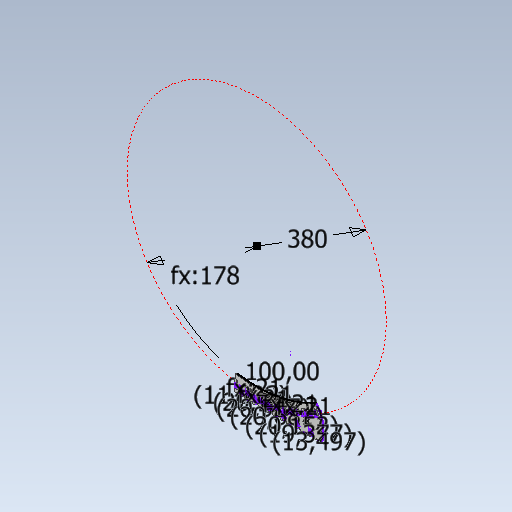
# Autodesk Inventor part: keywell_support-back
Saved by Autodesk Inventor 2020.1 (Build 241239000, 239)
## iProperties
Created: 2019-06-30
Part Number: keywell_support-back
Material: Acier inoxydable
Document SubType Name: Modeling
Designer: Thibault
Density: 8 g/cm^3
Appearance: Semi-poli
Mass: 13.686 g
Surface Area: 39.9351 cm^2
Volume: 1.71076 cm^3
kws_bp_anchor_dist1: 13,497 mm
kws_bp_anchor_dist2: 19,377 mm
kws_bp_anchor_dist3: 20,152 mm
kws_bp_anchor_dist4: 20,681 mm
kws_bp_anchor_dist5: 20,957 mm
kws_bp_anchor_dist6: 20,990 mm
kws_bp_anchor_dist7: 11,809 mm
Author: Thibault
Autodesk Inventor part; units mm, degrees
ref_plane "YZ Plane" through (0, 0, 0) normal (1, 0, 0) x (0, 1, 0)
ref_plane "XZ Plane" through (0, 0, 0) normal (0, 1, 0) x (-1, 0, 0)
ref_plane "XY Plane" through (0, 0, 0) normal (0, 0, 1) x (1, 0, 0)
sketch "Anchor (screw side)" plane through (0, 0, 0) normal (0, 0, 1) x (1, 0, 0)
  circle A0 centre (93.8994, 50.3042) radius 1.05
  line L0 (90.8494, 51.3542) -> (87.7494, 51.3542)
  line L1 (87.7494, 51.3542) -> (87.7494, 49.2542)
  line L2 (87.7494, 49.2542) -> (90.8494, 49.2542)
  line L3 (90.8494, 49.2542) -> (90.8494, 51.3542)
  line L4 (100.0494, 51.3542) -> (96.9494, 51.3542)
  line L5 (96.9494, 51.3542) -> (96.9494, 49.2542)
  line L6 (96.9494, 49.2542) -> (100.0494, 49.2542)
  line L7 (100.0494, 49.2542) -> (100.0494, 51.3542)
  line L8 (90.8494, 51.3542) -> (96.9494, 49.2542) construction
  line L9 (96.9494, 51.3542) -> (90.8494, 49.2542) construction
  line L10 (85.7494, 53.3542) -> (102.0494, 53.3542) construction
  line L11 (102.0494, 53.3542) -> (102.0494, 47.2542) construction
  line L12 (102.0494, 47.2542) -> (85.7494, 47.2542) construction
  line L13 (85.7494, 47.2542) -> (85.7494, 53.3542) construction
  point P0 (103.5798, 50.1132)
  dimension "d27" = 2.1
  dimension "d28" = 3.1
  dimension "d29" = 2.1
  dimension "slot_distance" = 6.1
  dimension "d34" = 2
  dimension "d35" = 2
  dimension "d36" = 2
  dimension "d37" = 2
  measures "d27" diameter of A0
  measures "d28" distance of L2.end L1.end
  measures "d29" distance of L1.end L0.end
  measures "slot_distance" distance between parallel lines of L5 L3
  measures "d34" distance between parallel lines of L0 L10
  measures "d35" distance between parallel lines of L12 L2
  measures "d36" distance between parallel lines of L11 L7
  measures "d37" distance between parallel lines of L13 L1
sketch "Anchor (nut side)" plane through (0, 0, 0) normal (0, 0, 1) x (1, 0, 0)
  line L0 (11.1, 0) -> (9.1, 0)
  line L1 (9.1, 0) -> (9.1, -2)
  line L2 (9.1, -2) -> (9.9, -2)
  line L3 (9.9, -2) -> (9.9, -4)
  line L4 (6.2, -4) -> (6.2, -2)
  line L5 (6.2, -2) -> (7, -2)
  line L6 (7, -2) -> (7, 0)
  line L7 (7, 0) -> (5, 0)
  line L8 (2, 0) -> (2, 2)
  line L9 (2, 0) -> (3, 0) construction
  line L10 (2, 2) -> (5, 2)
  line L11 (5, 2) -> (5, 0)
  line L12 (11.1, 0) -> (11.1, 2)
  line L13 (11.1, 2) -> (14.1, 2)
  line L14 (14.1, 2) -> (14.1, 0)
  line L15 (0, 0) -> (2, 0)
  line L16 (14.1, 0) -> (16.1, 0)
  line L17 (6.2, -4) -> (7, -4)
  line L18 (9.9, -4) -> (9.1, -4)
  line L19 (7, -4) -> (7, -6.25)
  line L20 (9.1, -4) -> (9.1, -6.25)
  line L21 (7.25, -6.5) -> (8.05, -6.5)
  arc A0 (7, -6.25) -> (7.25, -6.5) centre (7.25, -6.25) ccw
  arc A1 (8.85, -6.5) -> (9.1, -6.25) centre (8.85, -6.25) ccw
  line L22 (8.05, -6.5) -> (8.85, -6.5)
  line L23 (8.05, -3.8983) -> (8.05, -9.959) construction
  point P0 (9.1321, -0.6227)
  point P1 (7, -6.5)
  point P2 (9.1, -6.5)
  dimension "d3" = 2
  dimension "d7" = 6.1
  dimension "d10" = 2
  dimension "d11" = 2
  dimension "d12" = 0.8
  dimension "d13" = 2
  dimension "d14" = 0.8
  dimension "d15" = 2.1
  dimension "d18" = 2
  dimension "d19" = 0.8
  dimension "d20" = 0.8
  dimension "d21" = 2.5
  dimension "d22" = 2.5
  dimension "d23" = 2.1
  dimension "d38" = 2
  dimension "d39" = 0.25
  dimension "d120" = 3
  measures "d3" distance of point (0, 0) L8.start
  measures "d7" distance of L7.end L0.start
  measures "d10" distance of L0.start L0.end
  measures "d11" distance of L0.end L1.end
  measures "d12" distance of L1.end L2.end
  measures "d13" distance of L2.end L3.end
  measures "d14" distance of L4.end L5.end
  measures "d15" distance of L6.end L0.end
  measures "d18" distance of L14.end point (16.1, 0)
  measures "d19" distance of L4.start L17.end
  measures "d20" distance of L3.end L18.end
  measures "d21" distance of L17.end point (7, -6.5)
  measures "d22" distance of L18.end point (9.1, -6.5)
  measures "d23" distance of L17.end L18.end
  measures "d38" distance of the line from the sketch origin of L10
  measures "d39" radius of A0
  measures "d120" distance of L8.end L10.end
sketch "Screwless anchor (male)" plane through (0, 0, 0) normal (0, 0, 1) x (1, 0, 0)
  line L0 (2, 0) -> (2, 2)
  line L1 (2, 0) -> (3, 0) construction
  line L2 (2, 2) -> (5, 2)
  line L3 (5, 2) -> (5, 0)
  line L4 (11.1, 0) -> (11.1, 2)
  line L5 (11.1, 2) -> (14.1, 2)
  line L6 (14.1, 2) -> (14.1, 0)
  line L7 (0, 0) -> (2, 0)
  line L8 (14.1, 0) -> (16.1, 0)
  line L9 (5, 0) -> (11.1, 0)
  point P0 (9.1321, -0.6227)
  dimension "d81" = 2
  dimension "d83" = 6.1
  dimension "d92" = 2
  dimension "d100" = 2
  dimension "d119" = 3
  measures "d81" distance of L7.start L0.start
  measures "d83" distance of L3.end L4.start
  measures "d92" distance of L6.end L8.end
  measures "d100" distance between parallel lines of L7 L2
  measures "d119" distance of L0.end L2.end
sketch "Screwless anchor (female)" plane through (0, 0, 0) normal (0, 0, 1) x (1, 0, 0)
  line L0 (91.7814, 51.7592) -> (88.6814, 51.7592)
  line L1 (88.6814, 51.7592) -> (88.6814, 49.6592)
  line L2 (88.6814, 49.6592) -> (91.7814, 49.6592)
  line L3 (91.7814, 49.6592) -> (91.7814, 51.7592)
  line L4 (100.9814, 51.7592) -> (97.8814, 51.7592)
  line L5 (97.8814, 51.7592) -> (97.8814, 49.6592)
  line L6 (97.8814, 49.6592) -> (100.9814, 49.6592)
  line L7 (100.9814, 49.6592) -> (100.9814, 51.7592)
  line L8 (86.6814, 53.7592) -> (102.9814, 53.7592) construction
  line L9 (102.9814, 53.7592) -> (102.9814, 47.6592) construction
  line L10 (102.9814, 47.6592) -> (86.6814, 47.6592) construction
  line L11 (86.6814, 47.6592) -> (86.6814, 53.7592) construction
  point P0 (103.5798, 50.1132)
  dimension "d106" = 3.1
  dimension "d107" = 2.1
  dimension "d108" = 3.1
  dimension "d109" = 6.1
  dimension "d110" = 2
  dimension "d111" = 2
  dimension "d112" = 2
  dimension "d113" = 2
  measures "d106" distance of L2.end L1.end
  measures "d107" distance of L1.end L0.end
  measures "d108" distance of L6.end L5.end
  measures "d109" distance between parallel lines of L5 L3
  measures "d110" distance between parallel lines of L0 L8
  measures "d111" distance between parallel lines of L10 L2
  measures "d112" distance between parallel lines of L9 L7
  measures "d113" distance between parallel lines of L11 L1
sketch "Anchor" plane through (0, 0, 0) normal (0, 0, 1) x (1, 0, 0)
  line L0 (-55.968, -124.6471) -> (-43.668, -138.5471) construction
  line L1 (-43.668, -124.6471) -> (-55.968, -138.5471) construction
  line L2 (-49.818, -129.7478) -> (-49.818, -133.4207) construction
  circle A0 centre (-49.818, -123.5971) radius 1.05
  line L3 (-52.868, -122.5471) -> (-55.968, -122.5471)
  line L4 (-55.968, -122.5471) -> (-55.968, -124.6471)
  line L5 (-55.968, -124.6471) -> (-52.868, -124.6471)
  line L6 (-52.868, -124.6471) -> (-52.868, -122.5471)
  line L7 (-43.668, -122.5471) -> (-46.768, -122.5471)
  line L8 (-46.768, -122.5471) -> (-46.768, -124.6471)
  line L9 (-46.768, -124.6471) -> (-43.668, -124.6471)
  line L10 (-43.668, -124.6471) -> (-43.668, -122.5471)
  line L11 (-52.868, -122.5471) -> (-46.768, -124.6471) construction
  line L12 (-46.768, -122.5471) -> (-52.868, -124.6471) construction
  line L13 (-57.968, -120.5471) -> (-41.668, -120.5471) construction
  line L14 (-41.668, -120.5471) -> (-41.668, -126.6471) construction
  line L15 (-41.668, -126.6471) -> (-57.968, -126.6471) construction
  line L16 (-57.968, -126.6471) -> (-57.968, -120.5471) construction
  circle A1 centre (-49.818, -139.5971) radius 1.05
  line L17 (-52.868, -138.5471) -> (-55.968, -138.5471)
  line L18 (-55.968, -138.5471) -> (-55.968, -140.6471)
  line L19 (-55.968, -140.6471) -> (-52.868, -140.6471)
  line L20 (-52.868, -140.6471) -> (-52.868, -138.5471)
  line L21 (-43.668, -138.5471) -> (-46.768, -138.5471)
  line L22 (-46.768, -138.5471) -> (-46.768, -140.6471)
  line L23 (-46.768, -140.6471) -> (-43.668, -140.6471)
  line L24 (-43.668, -140.6471) -> (-43.668, -138.5471)
  line L25 (-52.868, -138.5471) -> (-46.768, -140.6471) construction
  line L26 (-46.768, -138.5471) -> (-52.868, -140.6471) construction
  line L27 (-57.968, -136.5471) -> (-41.668, -136.5471) construction
  line L28 (-41.668, -136.5471) -> (-41.668, -142.6471) construction
  line L29 (-41.668, -142.6471) -> (-57.968, -142.6471) construction
  line L30 (-57.968, -142.6471) -> (-57.968, -136.5471) construction
  point P0 (-66.8969, -206.6558)
  point P1 (-49.818, -123.5971)
  point P2 (-49.818, -139.5971)
  dimension "d161" = 13.9
sketch "Esquisse2" plane through (0, 0, 0) normal (0, 0, 1) x (1, 0, 0)
  circle A0 centre (0, 0) radius 190 construction
  arc A1 (-29.069, -175.6103) -> (87.3778, -155.0778) centre (0, 0) ccw
  line L0 (-31.1541, -195.9973) -> (-29.069, -175.6103)
  line L1 (49.6599, -108.8996) -> (49.6599, -114.6687) construction
  line L2 (96.3099, -173.5221) -> (96.3099, -198.7774)
  line L3 (-31.1541, -195.9973) -> (-31.1541, -198.7774)
  line L4 (30.8562, -181.468) -> (33.0699, -181.0776) construction
  line L5 (87.3778, -155.0778) -> (96.3099, -173.5221)
  line L6 (-27.395, -198.7774) -> (-31.1541, -198.7774)
  line L7 (-11.295, -198.7774) -> (-6.4051, -198.7774)
  line L8 (9.6949, -198.7774) -> (14.552, -198.7774)
  line L9 (30.652, -198.7774) -> (35.233, -198.7774)
  line L10 (51.333, -198.7774) -> (55.3852, -198.7774)
  line L11 (71.4852, -198.7774) -> (74.7625, -198.7774)
  line L12 (90.8625, -198.7774) -> (96.3099, -198.7774)
  line L13 (28.7711, -181.7178) -> (16.433, -195.584) construction
  line L14 (30.2343, -193.9304) -> (14.9698, -183.3713) construction
  line L15 (24.4382, -188.4309) -> (20.7913, -188.8678) construction
  circle A2 centre (30.5452, -187.6992) radius 1.05
  line L16 (31.2249, -184.546) -> (30.8562, -181.468)
  line L17 (30.8562, -181.468) -> (28.7711, -181.7178)
  line L18 (28.7711, -181.7178) -> (29.1398, -184.7958)
  line L19 (29.1398, -184.7958) -> (31.2249, -184.546)
  line L20 (32.3193, -193.6806) -> (31.9506, -190.6026)
  line L21 (31.9506, -190.6026) -> (29.8655, -190.8525)
  line L22 (29.8655, -190.8525) -> (30.2343, -193.9304)
  line L23 (30.2343, -193.9304) -> (32.3193, -193.6806)
  line L24 (31.2249, -184.546) -> (29.8655, -190.8525) construction
  line L25 (31.9506, -190.6026) -> (29.1398, -184.7958) construction
  line L26 (32.604, -179.2443) -> (34.5431, -195.4285) construction
  line L27 (34.5431, -195.4285) -> (28.4864, -196.1542) construction
  line L28 (28.4864, -196.1542) -> (26.5474, -179.9699) construction
  line L29 (26.5474, -179.9699) -> (32.604, -179.2443) construction
  circle A3 centre (14.6588, -189.6025) radius 1.05
  line L30 (15.3385, -186.4493) -> (14.9698, -183.3713)
  line L31 (14.9698, -183.3713) -> (12.8847, -183.6211)
  line L32 (12.8847, -183.6211) -> (13.2535, -186.6991)
  line L33 (13.2535, -186.6991) -> (15.3385, -186.4493)
  line L34 (16.433, -195.584) -> (16.0642, -192.506)
  line L35 (16.0642, -192.506) -> (13.9791, -192.7558)
  line L36 (13.9791, -192.7558) -> (14.3479, -195.8338)
  line L37 (14.3479, -195.8338) -> (16.433, -195.584)
  line L38 (15.3385, -186.4493) -> (13.9791, -192.7558) construction
  line L39 (16.0642, -192.506) -> (13.2535, -186.6991) construction
  line L40 (16.7177, -181.1476) -> (18.6567, -197.3318) construction
  line L41 (18.6567, -197.3318) -> (12.6, -198.0575) construction
  line L42 (12.6, -198.0575) -> (10.661, -181.8732) construction
  line L43 (10.661, -181.8732) -> (16.7177, -181.1476) construction
  line L44 (86.3871, -162.4389) -> (79.2379, -179.5675) construction
  line L45 (91.7481, -173.5091) -> (73.8769, -168.4973) construction
  line L46 (84.4769, -170.1971) -> (81.1712, -171.798) construction
  circle A4 centre (90.0126, -167.5164) radius 1.05
  line L47 (89.6283, -164.3137) -> (88.2771, -161.5236)
  line L48 (88.2771, -161.5236) -> (86.3871, -162.4389)
  line L49 (86.3871, -162.4389) -> (87.7382, -165.2289)
  line L50 (87.7382, -165.2289) -> (89.6283, -164.3137)
  line L51 (93.6381, -172.5938) -> (92.287, -169.8038)
  line L52 (92.287, -169.8038) -> (90.397, -170.7191)
  line L53 (90.397, -170.7191) -> (91.7481, -173.5091)
  line L54 (91.7481, -173.5091) -> (93.6381, -172.5938)
  line L55 (89.6283, -164.3137) -> (90.397, -170.7191) construction
  line L56 (92.287, -169.8038) -> (87.7382, -165.2289) construction
  line L57 (89.2055, -158.8519) -> (96.3099, -173.5221) construction
  line L58 (96.3099, -173.5221) -> (90.8198, -176.1808) construction
  line L59 (90.8198, -176.1808) -> (83.7154, -161.5106) construction
  line L60 (83.7154, -161.5106) -> (89.2055, -158.8519) construction
  circle A5 centre (75.6124, -174.49) radius 1.05
  line L61 (75.228, -171.2873) -> (73.8769, -168.4973)
  line L62 (73.8769, -168.4973) -> (71.9868, -169.4126)
  line L63 (71.9868, -169.4126) -> (73.338, -172.2026)
  line L64 (73.338, -172.2026) -> (75.228, -171.2873)
  line L65 (79.2379, -179.5675) -> (77.8867, -176.7774)
  line L66 (77.8867, -176.7774) -> (75.9967, -177.6927)
  line L67 (75.9967, -177.6927) -> (77.3478, -180.4828)
  line L68 (77.3478, -180.4828) -> (79.2379, -179.5675)
  line L69 (75.228, -171.2873) -> (75.9967, -177.6927) construction
  line L70 (77.8867, -176.7774) -> (73.338, -172.2026) construction
  line L71 (74.8052, -165.8255) -> (81.9096, -180.4958) construction
  line L72 (81.9096, -180.4958) -> (76.4195, -183.1545) construction
  line L73 (76.4195, -183.1545) -> (69.3151, -168.4843) construction
  line L74 (69.3151, -168.4843) -> (74.8052, -165.8255) construction
  line L75 (-5.2516, -196.2028) -> (8.5414, -183.7829) construction
  line L76 (-5.358, -183.9033) -> (8.6479, -196.0825) construction
  line L77 (-0.2043, -190.0089) -> (3.4685, -189.9771) construction
  circle A6 centre (-6.3548, -190.0621) radius 1.05
  line L78 (-7.3783, -193.1211) -> (-7.3515, -196.221)
  line L79 (-7.3515, -196.221) -> (-5.2516, -196.2028)
  line L80 (-5.2516, -196.2028) -> (-5.2784, -193.1029)
  line L81 (-5.2784, -193.1029) -> (-7.3783, -193.1211)
  line L82 (-7.458, -183.9215) -> (-7.4311, -187.0213)
  line L83 (-7.4311, -187.0213) -> (-5.3312, -187.0032)
  line L84 (-5.3312, -187.0032) -> (-5.358, -183.9033)
  line L85 (-5.358, -183.9033) -> (-7.458, -183.9215)
  line L86 (-7.3783, -193.1211) -> (-5.3312, -187.0032) construction
  line L87 (-7.4311, -187.0213) -> (-5.2784, -193.1029) construction
  line L88 (-9.3341, -198.2382) -> (-9.4752, -181.9389) construction
  line L89 (-9.4752, -181.9389) -> (-3.3754, -181.886) construction
  line L90 (-3.3754, -181.886) -> (-3.2343, -198.1854) construction
  line L91 (-3.2343, -198.1854) -> (-9.3341, -198.2382) construction
  circle A7 centre (9.6446, -189.9236) radius 1.05
  line L92 (8.6211, -192.9826) -> (8.6479, -196.0825)
  line L93 (8.6479, -196.0825) -> (10.7478, -196.0643)
  line L94 (10.7478, -196.0643) -> (10.721, -192.9644)
  line L95 (10.721, -192.9644) -> (8.6211, -192.9826)
  line L96 (8.5414, -183.7829) -> (8.5683, -186.8828)
  line L97 (8.5683, -186.8828) -> (10.6682, -186.8646)
  line L98 (10.6682, -186.8646) -> (10.6414, -183.7648)
  line L99 (10.6414, -183.7648) -> (8.5414, -183.7829)
  line L100 (8.6211, -192.9826) -> (10.6682, -186.8646) construction
  line L101 (8.5683, -186.8828) -> (10.721, -192.9644) construction
  line L102 (6.6653, -198.0997) -> (6.5242, -181.8003) construction
  line L103 (6.5242, -181.8003) -> (12.624, -181.7475) construction
  line L104 (12.624, -181.7475) -> (12.7651, -198.0469) construction
  line L105 (12.7651, -198.0469) -> (6.6653, -198.0997) construction
  line L106 (-26.8719, -194.4249) -> (-11.7926, -183.603) construction
  line L107 (-25.6204, -182.1887) -> (-13.0441, -195.8392) construction
  line L108 (-21.172, -188.8258) -> (-17.5181, -189.1995) construction
  circle A8 centre (-27.2907, -188.1999) radius 1.05
  line L109 (-28.6456, -191.1273) -> (-28.961, -194.2112)
  line L110 (-28.961, -194.2112) -> (-26.8719, -194.4249)
  line L111 (-26.8719, -194.4249) -> (-26.5565, -191.3409)
  line L112 (-26.5565, -191.3409) -> (-28.6456, -191.1273)
  line L113 (-27.7095, -181.975) -> (-28.0249, -185.0589)
  line L114 (-28.0249, -185.0589) -> (-25.9358, -185.2726)
  line L115 (-25.9358, -185.2726) -> (-25.6204, -182.1887)
  line L116 (-25.6204, -182.1887) -> (-27.7095, -181.975)
  line L117 (-28.6456, -191.1273) -> (-25.9358, -185.2726) construction
  line L118 (-28.0249, -185.0589) -> (-26.5565, -191.3409) construction
  line L119 (-31.1541, -195.9973) -> (-29.4956, -179.7819) construction
  line L120 (-29.4956, -179.7819) -> (-23.4273, -180.4026) construction
  line L121 (-23.4273, -180.4026) -> (-25.0858, -196.618) construction
  line L122 (-25.0858, -196.618) -> (-31.1541, -195.9973) construction
  circle A9 centre (-11.3738, -189.8279) radius 1.05
  line L123 (-12.7286, -192.7553) -> (-13.0441, -195.8392)
  line L124 (-13.0441, -195.8392) -> (-10.955, -196.0528)
  line L125 (-10.955, -196.0528) -> (-10.6395, -192.9689)
  line L126 (-10.6395, -192.9689) -> (-12.7286, -192.7553)
  line L127 (-11.7926, -183.603) -> (-12.108, -186.6869)
  line L128 (-12.108, -186.6869) -> (-10.0189, -186.9006)
  line L129 (-10.0189, -186.9006) -> (-9.7034, -183.8167)
  line L130 (-9.7034, -183.8167) -> (-11.7926, -183.603)
  line L131 (-12.7286, -192.7553) -> (-10.0189, -186.9006) construction
  line L132 (-12.108, -186.6869) -> (-10.6395, -192.9689) construction
  line L133 (-15.2372, -197.6253) -> (-13.5787, -181.4099) construction
  line L134 (-13.5787, -181.4099) -> (-7.5103, -182.0305) construction
  line L135 (-7.5103, -182.0305) -> (-9.1688, -198.246) construction
  line L136 (-9.1688, -198.246) -> (-15.2372, -197.6253) construction
  line L137 (48.6492, -177.4327) -> (37.9167, -192.5758) construction
  line L138 (51.4512, -189.4093) -> (35.1147, -180.5992) construction
  line L139 (45.0837, -184.583) -> (41.5073, -185.4197) construction
  circle A10 centre (51.0726, -183.1818) radius 1.05
  line L140 (51.4002, -179.9728) -> (50.694, -176.9543)
  line L141 (50.694, -176.9543) -> (48.6492, -177.4327)
  line L142 (48.6492, -177.4327) -> (49.3554, -180.4512)
  line L143 (49.3554, -180.4512) -> (51.4002, -179.9728)
  line L144 (53.496, -188.9309) -> (52.7898, -185.9125)
  line L145 (52.7898, -185.9125) -> (50.745, -186.3908)
  line L146 (50.745, -186.3908) -> (51.4512, -189.4093)
  line L147 (51.4512, -189.4093) -> (53.496, -188.9309)
  line L148 (51.4002, -179.9728) -> (50.745, -186.3908) construction
  line L149 (52.7898, -185.9125) -> (49.3554, -180.4512) construction
  line L150 (52.1858, -174.5513) -> (55.899, -190.4227) construction
  line L151 (55.899, -190.4227) -> (49.9594, -191.8124) construction
  line L152 (49.9594, -191.8124) -> (46.2462, -175.9409) construction
  line L153 (46.2462, -175.9409) -> (52.1858, -174.5513) construction
  circle A11 centre (35.4933, -186.8267) radius 1.05
  line L154 (35.8209, -183.6177) -> (35.1147, -180.5992)
  line L155 (35.1147, -180.5992) -> (33.0699, -181.0776)
  line L156 (33.0699, -181.0776) -> (33.7761, -184.0961)
  line L157 (33.7761, -184.0961) -> (35.8209, -183.6177)
  line L158 (37.9167, -192.5758) -> (37.2105, -189.5573)
  line L159 (37.2105, -189.5573) -> (35.1657, -190.0357)
  line L160 (35.1657, -190.0357) -> (35.8719, -193.0542)
  line L161 (35.8719, -193.0542) -> (37.9167, -192.5758)
  line L162 (35.8209, -183.6177) -> (35.1657, -190.0357) construction
  line L163 (37.2105, -189.5573) -> (33.7761, -184.0961) construction
  line L164 (36.6065, -178.1962) -> (40.3197, -194.0676) construction
  line L165 (40.3197, -194.0676) -> (34.3801, -195.4572) construction
  line L166 (34.3801, -195.4572) -> (30.6669, -179.5858) construction
  line L167 (30.6669, -179.5858) -> (36.6065, -178.1962) construction
  line L168 (67.9331, -170.9802) -> (58.9373, -187.2152) construction
  line L169 (72.0397, -182.5744) -> (54.8307, -175.621) construction
  line L170 (65.1784, -178.4802) -> (61.7162, -179.7065) construction
  circle A12 centre (70.9762, -176.4267) radius 1.05
  line L171 (70.9476, -173.2012) -> (69.9126, -170.279)
  line L172 (69.9126, -170.279) -> (67.9331, -170.9802)
  line L173 (67.9331, -170.9802) -> (68.9681, -173.9023)
  line L174 (68.9681, -173.9023) -> (70.9476, -173.2012)
  line L175 (74.0192, -181.8733) -> (72.9842, -178.9511)
  line L176 (72.9842, -178.9511) -> (71.0047, -179.6523)
  line L177 (71.0047, -179.6523) -> (72.0397, -182.5744)
  line L178 (72.0397, -182.5744) -> (74.0192, -181.8733)
  line L179 (70.9476, -173.2012) -> (71.0047, -179.6523) construction
  line L180 (72.9842, -178.9511) -> (68.9681, -173.9023) construction
  line L181 (71.1301, -167.7261) -> (76.5722, -183.0908) construction
  line L182 (76.5722, -183.0908) -> (70.8222, -185.1274) construction
  line L183 (70.8222, -185.1274) -> (65.3801, -169.7627) construction
  line L184 (65.3801, -169.7627) -> (71.1301, -167.7261) construction
  circle A13 centre (55.8942, -181.7686) radius 1.05
  line L185 (55.8657, -178.5431) -> (54.8307, -175.621)
  line L186 (54.8307, -175.621) -> (52.8512, -176.3221)
  line L187 (52.8512, -176.3221) -> (53.8862, -179.2442)
  line L188 (53.8862, -179.2442) -> (55.8657, -178.5431)
  line L189 (58.9373, -187.2152) -> (57.9023, -184.2931)
  line L190 (57.9023, -184.2931) -> (55.9228, -184.9942)
  line L191 (55.9228, -184.9942) -> (56.9578, -187.9163)
  line L192 (56.9578, -187.9163) -> (58.9373, -187.2152)
  line L193 (55.8657, -178.5431) -> (55.9228, -184.9942) construction
  line L194 (57.9023, -184.2931) -> (53.8862, -179.2442) construction
  line L195 (56.0482, -173.068) -> (61.4903, -188.4327) construction
  line L196 (61.4903, -188.4327) -> (55.7403, -190.4693) construction
  line L197 (55.7403, -190.4693) -> (50.2982, -175.1046) construction
  line L198 (50.2982, -175.1046) -> (56.0482, -173.068) construction
  line L199 (-22.395, -198.7774) -> (-20.395, -198.7774)
  line L200 (-20.395, -198.7774) -> (-20.395, -196.7774)
  line L201 (-20.395, -196.7774) -> (-21.195, -196.7774)
  line L202 (-21.195, -196.7774) -> (-21.195, -194.7774)
  line L203 (-17.495, -194.7774) -> (-17.495, -196.7774)
  line L204 (-17.495, -196.7774) -> (-18.295, -196.7774)
  line L205 (-18.295, -196.7774) -> (-18.295, -198.7774)
  line L206 (-18.295, -198.7774) -> (-16.295, -198.7774)
  line L207 (-13.295, -198.7774) -> (-13.295, -200.7774)
  line L208 (-13.295, -198.7774) -> (-14.295, -198.7774) construction
  line L209 (-13.295, -200.7774) -> (-16.295, -200.7774)
  line L210 (-16.295, -200.7774) -> (-16.295, -198.7774)
  line L211 (-22.395, -198.7774) -> (-22.395, -200.7774)
  line L212 (-22.395, -200.7774) -> (-25.395, -200.7774)
  line L213 (-25.395, -200.7774) -> (-25.395, -198.7774)
  line L214 (-11.295, -198.7774) -> (-13.295, -198.7774)
  line L215 (-25.395, -198.7774) -> (-27.395, -198.7774)
  line L216 (-17.495, -194.7774) -> (-18.295, -194.7774)
  line L217 (-21.195, -194.7774) -> (-20.395, -194.7774)
  line L218 (-18.295, -194.7774) -> (-18.295, -192.5274)
  line L219 (-20.395, -194.7774) -> (-20.395, -192.5274)
  line L220 (-18.545, -192.2774) -> (-19.345, -192.2774)
  arc A14 (-18.295, -192.5274) -> (-18.545, -192.2774) centre (-18.545, -192.5274) ccw
  arc A15 (-20.145, -192.2774) -> (-20.395, -192.5274) centre (-20.145, -192.5274) ccw
  line L221 (-19.345, -192.2774) -> (-20.145, -192.2774)
  line L222 (-19.345, -194.8792) -> (-19.345, -188.8184) construction
  line L223 (-1.4051, -198.7774) -> (0.5949, -198.7774)
  line L224 (0.5949, -198.7774) -> (0.5949, -196.7774)
  line L225 (0.5949, -196.7774) -> (-0.2051, -196.7774)
  line L226 (-0.2051, -196.7774) -> (-0.2051, -194.7774)
  line L227 (3.4949, -194.7774) -> (3.4949, -196.7774)
  line L228 (3.4949, -196.7774) -> (2.6949, -196.7774)
  line L229 (2.6949, -196.7774) -> (2.6949, -198.7774)
  line L230 (2.6949, -198.7774) -> (4.6949, -198.7774)
  line L231 (7.6949, -198.7774) -> (7.6949, -200.7774)
  line L232 (7.6949, -198.7774) -> (6.6949, -198.7774) construction
  line L233 (7.6949, -200.7774) -> (4.6949, -200.7774)
  line L234 (4.6949, -200.7774) -> (4.6949, -198.7774)
  line L235 (-1.4051, -198.7774) -> (-1.4051, -200.7774)
  line L236 (-1.4051, -200.7774) -> (-4.4051, -200.7774)
  line L237 (-4.4051, -200.7774) -> (-4.4051, -198.7774)
  line L238 (9.6949, -198.7774) -> (7.6949, -198.7774)
  line L239 (-4.4051, -198.7774) -> (-6.4051, -198.7774)
  line L240 (3.4949, -194.7774) -> (2.6949, -194.7774)
  line L241 (-0.2051, -194.7774) -> (0.5949, -194.7774)
  line L242 (2.6949, -194.7774) -> (2.6949, -192.5274)
  line L243 (0.5949, -194.7774) -> (0.5949, -192.5274)
  line L244 (2.4449, -192.2774) -> (1.6449, -192.2774)
  arc A16 (2.6949, -192.5274) -> (2.4449, -192.2774) centre (2.4449, -192.5274) ccw
  arc A17 (0.8449, -192.2774) -> (0.5949, -192.5274) centre (0.8449, -192.5274) ccw
  line L245 (1.6449, -192.2774) -> (0.8449, -192.2774)
  line L246 (1.6449, -194.8792) -> (1.6449, -188.8184) construction
  line L247 (19.552, -198.7774) -> (21.552, -198.7774)
  line L248 (21.552, -198.7774) -> (21.552, -196.7774)
  line L249 (21.552, -196.7774) -> (20.752, -196.7774)
  line L250 (20.752, -196.7774) -> (20.752, -194.7774)
  line L251 (24.452, -194.7774) -> (24.452, -196.7774)
  line L252 (24.452, -196.7774) -> (23.652, -196.7774)
  line L253 (23.652, -196.7774) -> (23.652, -198.7774)
  line L254 (23.652, -198.7774) -> (25.652, -198.7774)
  line L255 (28.652, -198.7774) -> (28.652, -200.7774)
  line L256 (28.652, -198.7774) -> (27.652, -198.7774) construction
  line L257 (28.652, -200.7774) -> (25.652, -200.7774)
  line L258 (25.652, -200.7774) -> (25.652, -198.7774)
  line L259 (19.552, -198.7774) -> (19.552, -200.7774)
  line L260 (19.552, -200.7774) -> (16.552, -200.7774)
  line L261 (16.552, -200.7774) -> (16.552, -198.7774)
  line L262 (30.652, -198.7774) -> (28.652, -198.7774)
  line L263 (16.552, -198.7774) -> (14.552, -198.7774)
  line L264 (24.452, -194.7774) -> (23.652, -194.7774)
  line L265 (20.752, -194.7774) -> (21.552, -194.7774)
  line L266 (23.652, -194.7774) -> (23.652, -192.5274)
  line L267 (21.552, -194.7774) -> (21.552, -192.5274)
  line L268 (23.402, -192.2774) -> (22.602, -192.2774)
  arc A18 (23.652, -192.5274) -> (23.402, -192.2774) centre (23.402, -192.5274) ccw
  arc A19 (21.802, -192.2774) -> (21.552, -192.5274) centre (21.802, -192.5274) ccw
  line L269 (22.602, -192.2774) -> (21.802, -192.2774)
  line L270 (22.602, -194.8792) -> (22.602, -188.8184) construction
  line L271 (40.233, -198.7774) -> (42.233, -198.7774)
  line L272 (42.233, -198.7774) -> (42.233, -196.7774)
  line L273 (42.233, -196.7774) -> (41.433, -196.7774)
  line L274 (41.433, -196.7774) -> (41.433, -194.7774)
  line L275 (45.133, -194.7774) -> (45.133, -196.7774)
  line L276 (45.133, -196.7774) -> (44.333, -196.7774)
  line L277 (44.333, -196.7774) -> (44.333, -198.7774)
  line L278 (44.333, -198.7774) -> (46.333, -198.7774)
  line L279 (49.333, -198.7774) -> (49.333, -200.7774)
  line L280 (49.333, -198.7774) -> (48.333, -198.7774) construction
  line L281 (49.333, -200.7774) -> (46.333, -200.7774)
  line L282 (46.333, -200.7774) -> (46.333, -198.7774)
  line L283 (40.233, -198.7774) -> (40.233, -200.7774)
  line L284 (40.233, -200.7774) -> (37.233, -200.7774)
  line L285 (37.233, -200.7774) -> (37.233, -198.7774)
  line L286 (51.333, -198.7774) -> (49.333, -198.7774)
  line L287 (37.233, -198.7774) -> (35.233, -198.7774)
  line L288 (45.133, -194.7774) -> (44.333, -194.7774)
  line L289 (41.433, -194.7774) -> (42.233, -194.7774)
  line L290 (44.333, -194.7774) -> (44.333, -192.5274)
  line L291 (42.233, -194.7774) -> (42.233, -192.5274)
  line L292 (44.083, -192.2774) -> (43.283, -192.2774)
  arc A20 (44.333, -192.5274) -> (44.083, -192.2774) centre (44.083, -192.5274) ccw
  arc A21 (42.483, -192.2774) -> (42.233, -192.5274) centre (42.483, -192.5274) ccw
  line L293 (43.283, -192.2774) -> (42.483, -192.2774)
  line L294 (43.283, -194.8792) -> (43.283, -188.8184) construction
  line L295 (60.3852, -198.7774) -> (62.3852, -198.7774)
  line L296 (62.3852, -198.7774) -> (62.3852, -196.7774)
  line L297 (62.3852, -196.7774) -> (61.5852, -196.7774)
  line L298 (61.5852, -196.7774) -> (61.5852, -194.7774)
  line L299 (65.2852, -194.7774) -> (65.2852, -196.7774)
  line L300 (65.2852, -196.7774) -> (64.4852, -196.7774)
  line L301 (64.4852, -196.7774) -> (64.4852, -198.7774)
  line L302 (64.4852, -198.7774) -> (66.4852, -198.7774)
  line L303 (69.4852, -198.7774) -> (69.4852, -200.7774)
  line L304 (69.4852, -198.7774) -> (68.4852, -198.7774) construction
  line L305 (69.4852, -200.7774) -> (66.4852, -200.7774)
  line L306 (66.4852, -200.7774) -> (66.4852, -198.7774)
  line L307 (60.3852, -198.7774) -> (60.3852, -200.7774)
  line L308 (60.3852, -200.7774) -> (57.3852, -200.7774)
  line L309 (57.3852, -200.7774) -> (57.3852, -198.7774)
  line L310 (71.4852, -198.7774) -> (69.4852, -198.7774)
  line L311 (57.3852, -198.7774) -> (55.3852, -198.7774)
  line L312 (65.2852, -194.7774) -> (64.4852, -194.7774)
  line L313 (61.5852, -194.7774) -> (62.3852, -194.7774)
  line L314 (64.4852, -194.7774) -> (64.4852, -192.5274)
  line L315 (62.3852, -194.7774) -> (62.3852, -192.5274)
  line L316 (64.2352, -192.2774) -> (63.4352, -192.2774)
  arc A22 (64.4852, -192.5274) -> (64.2352, -192.2774) centre (64.2352, -192.5274) ccw
  arc A23 (62.6352, -192.2774) -> (62.3852, -192.5274) centre (62.6352, -192.5274) ccw
  line L317 (63.4352, -192.2774) -> (62.6352, -192.2774)
  line L318 (63.4352, -194.8792) -> (63.4352, -188.8184) construction
  line L319 (79.7625, -198.7774) -> (81.7625, -198.7774)
  line L320 (81.7625, -198.7774) -> (81.7625, -196.7774)
  line L321 (81.7625, -196.7774) -> (80.9625, -196.7774)
  line L322 (80.9625, -196.7774) -> (80.9625, -194.7774)
  line L323 (84.6625, -194.7774) -> (84.6625, -196.7774)
  line L324 (84.6625, -196.7774) -> (83.8625, -196.7774)
  line L325 (83.8625, -196.7774) -> (83.8625, -198.7774)
  line L326 (83.8625, -198.7774) -> (85.8625, -198.7774)
  line L327 (88.8625, -198.7774) -> (88.8625, -200.7774)
  line L328 (88.8625, -198.7774) -> (87.8625, -198.7774) construction
  line L329 (88.8625, -200.7774) -> (85.8625, -200.7774)
  line L330 (85.8625, -200.7774) -> (85.8625, -198.7774)
  line L331 (79.7625, -198.7774) -> (79.7625, -200.7774)
  line L332 (79.7625, -200.7774) -> (76.7625, -200.7774)
  line L333 (76.7625, -200.7774) -> (76.7625, -198.7774)
  line L334 (90.8625, -198.7774) -> (88.8625, -198.7774)
  line L335 (76.7625, -198.7774) -> (74.7625, -198.7774)
  line L336 (84.6625, -194.7774) -> (83.8625, -194.7774)
  line L337 (80.9625, -194.7774) -> (81.7625, -194.7774)
  line L338 (83.8625, -194.7774) -> (83.8625, -192.5274)
  line L339 (81.7625, -194.7774) -> (81.7625, -192.5274)
  line L340 (83.6125, -192.2774) -> (82.8125, -192.2774)
  arc A24 (83.8625, -192.5274) -> (83.6125, -192.2774) centre (83.6125, -192.5274) ccw
  arc A25 (82.0125, -192.2774) -> (81.7625, -192.5274) centre (82.0125, -192.5274) ccw
  line L341 (82.8125, -192.2774) -> (82.0125, -192.2774)
  line L342 (82.8125, -194.8792) -> (82.8125, -188.8184) construction
  point P0 (1.6449, -189.9929)
  point P1 (-19.3322, -189.0139)
  point P2 (43.283, -185.0043)
  point P3 (63.4352, -179.0977)
  point P4 (22.602, -188.6509)
  point P5 (82.8125, -171.0032)
  point P6 (-19.3322, -189.0139)
  point P7 (1.6449, -189.9929)
  point P8 (22.602, -188.6509)
  point P9 (63.4352, -179.0977)
  point P10 (82.8125, -171.0032)
  point P11 (82.8125, -171.0032)
  point P12 (63.4352, -179.0977)
  point P13 (43.283, -185.0043)
  point P14 (22.602, -188.6509)
  point P15 (1.6449, -189.9929)
  point P16 (-19.345, -189.0126)
  dimension "kws_bp_anchor_dist2" = 19.3773
  dimension "kws_bp_anchor_dist3" = 20.1522
  dimension "kws_bp_anchor_dist4" = 20.681
  dimension "kws_bp_anchor_dist5" = 20.9571
  dimension "kws_bp_anchor_dist6" = 20.99
  dimension "radius" = 380
  dimension "d73" = 178
  dimension "d163" = 21
  dimension "d164" = 21
  dimension "d165" = 21
  dimension "d166" = 21
  dimension "d167" = 21
  dimension "d170" = 80
  dimension "kws_bp_anchor_dist1" = 13.4974
  dimension "kws_bp_anchor_dist7" = 11.8091
  constraints: 26 end point, 8 point on circle, 7 horizontal, 3 vertical, 2 centre point, 1 coincident, 49 other
  measures "radius" diameter of A0
  measures "d73" radius of A1
  measures "d163" distance of A0.start A0.end
  measures "d164" distance of point (22.602, -188.651) point (43.283, -185.004)
  measures "d165" distance of point (43.283, -185.004) point (63.435, -179.098)
  measures "d166" distance of point (63.435, -179.098) point (82.812, -171.003)
  measures "d167" distance of A0.start point (22.602, -188.651)
  measures "d170" angle of L4 L1
extrude "Base" add sketch "Esquisse2" along normal blind 2
sketch "Esquisse5" plane through (0, 0, 2) normal (0, 0, 1) x (1, 0, 0)
  line L0 (50.0053, -108.084) -> (185.8962, -108.084)
  line L1 (185.8962, -108.084) -> (185.8962, -257.6603)
  line L2 (50.0053, -108.084) -> (76.5722, -183.0908)
  line L3 (76.5722, -183.0908) -> (76.5722, -257.6603)
  line L4 (76.5722, -257.6603) -> (185.8962, -257.6603)
  line L5 (69.9126, -170.279) -> (70.9476, -173.2012) projected
  line L6 (74.0192, -181.8733) -> (72.0397, -182.5744) projected
  point P0 (0, 0)
  dimension "d171" = 2
  dimension "d172" = 2
  constraints: 10 end point, 2 perpendicular, 1 horizontal, 1 parallel, 1 vertical
  measures "d171" distance between parallel lines of L5 L2
  measures "d172" distance from line of L2.end L6
extrude "Front: substract" [suppressed]
sketch "Esquisse7" plane through (0, 0, 2) normal (0, 0, 1) x (1, 0, 0)
  line L0 (74.6869, -183.7585) -> (56.1294, -131.3647)
  line L1 (72.5845, -177.8226) -> (73.002, -179.0013)
  line L2 (-107.3318, -264.8349) -> (-95.7555, -119.2846)
  line L3 (-95.7555, -119.2846) -> (56.1294, -131.3647)
  line L4 (74.6869, -183.7585) -> (74.6869, -264.8349)
  line L5 (74.6869, -264.8349) -> (-107.3318, -264.8349)
  line L6 (73.338, -172.2026) -> (71.9868, -169.4126) projected
  line L7 (69.9126, -170.279) -> (70.9476, -173.2012) projected
  line L8 (74.0192, -181.8733) -> (72.0397, -182.5744) projected
  point P0 (0, 0)
  dimension "d175" = 2
  constraints: 12 end point, 2 collinear, 2 perpendicular, 1 vertical
  measures "d175" distance from line of L0.start L8
extrude "Front r6: substract" [suppressed]
derived "shared_parameters.ipt"
sketch "Esquisse9" plane through (0, 0, 2) normal (0, 0, 1) x (1, 0, 0)
  line L0 (90.8625, -176.1602) -> (174.0508, -135.8742)
  line L1 (93.6381, -172.5938) -> (91.7481, -173.5091) projected
  line L2 (90.8625, -176.1602) -> (90.8625, -265.0205)
  line L3 (88.8625, -200.7774) -> (88.8625, -198.7774) projected
  line L4 (174.0508, -135.8742) -> (174.0508, -265.0205)
  line L5 (174.0508, -265.0205) -> (90.8625, -265.0205)
  point P0 (0, 0)
  dimension "d192" = 2
  dimension "d193" = 2
  constraints: 9 end point, 2 vertical, 1 parallel, 1 perpendicular
  measures "d192" distance between parallel lines of L0 L1
  measures "d193" distance between parallel lines of L2 L3
extrude "Gain de place" [suppressed]
equation "\"esd\" = 0.1"
